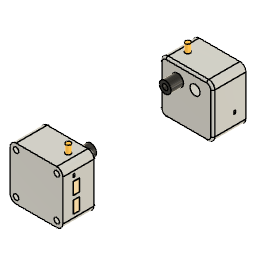
Final design 2025 project v9 (Autodesk Fusion 360 design; units mm, degrees)
Autodesk Fusion 360 part; units mm, degrees
note: some values were not read from the file. Chosen so that the rebuilt part matches the saved one: which bodies a step acts on. Set by a fixed rule: which sketch regions a step uses.
(part 1 of 2)
sketch "Sketch1" plane through (0, 0, 0) normal (0, 1, 0) x (1, 0, 0)
  line L0 (4, 0) -> (53, 0)
  line L1 (57, -4) -> (57, -53)
  line L2 (53, -57) -> (4, -57)
  line L3 (0, -53) -> (0, -4)
  circle A0 centre (18, -43.5) radius 8
  circle A1 centre (39, -43.5) radius 8
  arc A2 (0, -53) -> (4, -57) centre (4, -53) ccw
  arc A3 (53, -57) -> (57, -53) centre (53, -53) ccw
  arc A4 (57, -4) -> (53, 0) centre (53, -4) ccw
  arc A5 (4, 0) -> (0, -4) centre (4, -4) ccw
  circle A6 centre (18, -43.5) radius 2.8
  circle A7 centre (39, -43.5) radius 2.8
  circle A8 centre (4, -53) radius 1.8
  circle A9 centre (53, -53) radius 1.8
  circle A10 centre (4, -4) radius 1.8
  circle A11 centre (53, -4) radius 1.8
  line L4 (0, -8) -> (11.1, -8)
  line L5 (11.1, -8) -> (11.1, -22.6)
  line L6 (11.1, -22.6) -> (0, -22.6)
  line L7 (0, -22.6) -> (0, -8)
  line L8 (0, -27.6) -> (11.1, -27.6)
  line L9 (11.1, -27.6) -> (11.1, -42.2)
  line L10 (11.1, -42.2) -> (0, -42.2)
  line L11 (0, -42.2) -> (0, -27.6)
  line L12 (10, -57) -> (14.9, -57)
  line L13 (14.9, -57) -> (14.9, -47.5)
  line L14 (14.9, -47.5) -> (10, -47.5)
  line L15 (10, -47.5) -> (10, -57)
  line L16 (0, -49) -> (1, -49)
  line L17 (1, -49) -> (1, -47)
  line L18 (1, -47) -> (0, -47)
  line L19 (0, -47) -> (0, -49)
  arc A12 (-0.8, -53) -> (4, -57.8) centre (4, -53) ccw
  line L20 (53, -57.8) -> (4, -57.8)
  arc A13 (53, -57.8) -> (57.8, -53) centre (53, -53) ccw
  line L21 (57.8, -4) -> (57.8, -53)
  arc A14 (57.8, -4) -> (53, 0.8) centre (53, -4) ccw
  line L22 (4, 0.8) -> (53, 0.8)
  arc A15 (4, 0.8) -> (-0.8, -4) centre (4, -4) ccw
  line L23 (-0.8, -53) -> (-0.8, -4)
  arc A16 (-3.3, -53) -> (4, -60.3) centre (4, -53) ccw
  line L24 (53, -60.3) -> (4, -60.3)
  arc A17 (53, -60.3) -> (60.3, -53) centre (53, -53) ccw
  line L25 (60.3, -4) -> (60.3, -53)
  arc A18 (60.3, -4) -> (53, 3.3) centre (53, -4) ccw
  line L26 (4, 3.3) -> (53, 3.3)
  arc A19 (4, 3.3) -> (-3.3, -4) centre (4, -4) ccw
  line L27 (-3.3, -53) -> (-3.3, -4)
  arc A20 (0.6, -53) -> (4, -56.4) centre (4, -53) ccw
  line L28 (53, -56.4) -> (4, -56.4)
  arc A21 (53, -56.4) -> (56.4, -53) centre (53, -53) ccw
  line L29 (56.4, -4) -> (56.4, -53)
  arc A22 (56.4, -4) -> (53, -0.6) centre (53, -4) ccw
  line L30 (4, -0.6) -> (53, -0.6)
  arc A23 (4, -0.6) -> (0.6, -4) centre (4, -4) ccw
  line L31 (0.6, -53) -> (0.6, -4)
  arc A24 (0.8, -53) -> (4, -56.2) centre (4, -53) ccw
  line L32 (53, -56.2) -> (4, -56.2)
  arc A25 (53, -56.2) -> (56.2, -53) centre (53, -53) ccw
  line L33 (56.2, -4) -> (56.2, -53)
  arc A26 (56.2, -4) -> (53, -0.8) centre (53, -4) ccw
  line L34 (4, -0.8) -> (53, -0.8)
  arc A27 (4, -0.8) -> (0.8, -4) centre (4, -4) ccw
  line L35 (0.8, -53) -> (0.8, -4)
  line L36 (60.3, -20.1347) -> (60.3, -16.7)
  line L37 (56.2, -16.7) -> (55.2, -16.7)
  line L38 (55.2, -16.7) -> (55.2, -18.7)
  line L39 (55.2, -18.7) -> (56.2, -18.7)
  line L40 (56.2, -18.7) -> (56.2, -16.7)
  line L41 (9.43, -57) -> (13.43, -57)
  line L42 (13.43, -57) -> (13.43, -55)
  line L43 (13.43, -55) -> (9.43, -55)
  line L44 (9.43, -55) -> (9.43, -57)
  point P0 (57, 0)
  point P1 (0, -57)
  dimension "d1" = 57
  dimension "d2" = 57
  dimension "d13" = 16
  dimension "d15" = 16
  dimension "d16" = 4
  dimension "d17" = 5.6
  dimension "d18" = 5.6
  dimension "d21" = 3.6
  dimension "d22" = 3.6
  dimension "d23" = 3.6
  dimension "d24" = 3.6
  dimension "d29" = 11.1
  dimension "d30" = 11.1
  dimension "d31" = 14.6
  dimension "d34" = 4.9
  dimension "d35" = 9.5
  dimension "d37" = 1
  dimension "d38" = 2
  dimension "d40" = -0.8
  dimension "d41" = -2.5
  dimension "d58" = 0.6
  dimension "d59" = 0.8
  dimension "d61" = 1
  dimension "d62" = 2
  dimension "d65" = 4
  dimension "d66" = 2
  constraint horizontal L0
  constraint vertical L1
  constraint horizontal L2
  constraint vertical L3
  constraint coincident P1 L2
  constraint coincident P1 L3
  constraint tangent L2 A2
  constraint tangent L3 A2
  constraint tangent L1 A3
  constraint tangent L2 A3
  constraint equal A2 A3
  constraint coincident P0 L0
  constraint coincident P0 L1
  constraint tangent L0 A4
  constraint tangent L1 A4
  constraint equal A2 A4
  constraint coincident origin L0
  constraint coincident origin L3
  constraint tangent L0 A5
  constraint tangent L3 A5
  constraint equal A2 A5
  constraint concentric A0 A6
  constraint concentric A1 A7
  constraint concentric A2 A8
  constraint concentric A3 A9
  constraint concentric A5 A10
  constraint concentric A4 A11
  constraint horizontal L4
  constraint vertical L5
  constraint horizontal L6
  constraint vertical L7
  constraint horizontal L8
  constraint vertical L9
  constraint horizontal L10
  constraint vertical L11
  constraint horizontal L12
  constraint vertical L13
  constraint horizontal L14
  constraint vertical L15
  constraint coincident L2 L12.start
  constraint horizontal L16
  constraint vertical L17
  constraint horizontal L18
  constraint vertical L19
  constraint coincident L3 L16.start
  constraint vertical L36
  constraint coincident L25 L36.end
  constraint horizontal L37
  constraint vertical L38
  constraint horizontal L39
  constraint vertical L40
  constraint coincident L33 L37.start
  constraint horizontal L41
  constraint vertical L42
  constraint horizontal L43
  constraint vertical L44
  constraint coincident L2 L41.start
  measures "d1" distance of origin P0
  measures "d2" distance of origin P1
  measures "d13" diameter of A0
  measures "d15" diameter of A1
  measures "d16" radius of A2
  measures "d17" diameter of A6
  measures "d18" diameter of A7
  measures "d21" diameter of A8
  measures "d22" diameter of A9
  measures "d23" diameter of A10
  measures "d24" diameter of A11
  measures "d29" distance of L4.start L4.end
  measures "d30" distance of L8.start L8.end
  measures "d31" distance of L8.start L10.end
  measures "d34" distance of L12.start L12.end
  measures "d35" distance of L12.start L14.end
  measures "d37" distance of L16.start L16.end
  measures "d38" distance of L16.start L18.end
  measures "d61" distance of L37.start L37.end
  measures "d62" distance of L37.start L39.end
  measures "d65" distance of L41.start L41.end
  measures "d66" distance of L41.start L43.end
extrude "Extrude7" add sketch "Sketch1" along normal blind 1 contours L0 L1 L2 L3 A3 A4 A5 L4 L13 L28 A21 L29 A22 L30 A23 L31 | L3 L6 L8 L31 | L4 L13 L28 A21 L29 A22 L30 A23 L31 L32 A25 L33 A26 L34 A27 L35 L40 | L4 L6 L31 L35 | L6 L8 L31 L35 | A0 L4 L5 L6 L8 L9 L13 L32 A25 L33 A26 L34 A27 L35 L37 L38 L39 | L4 L5 L6 L35 | L2 L12 L13 L28 L42 | L3 L10 L18 L31 | L8 L10 L31 L35 | L13 L28 L32 L42 | L10 L18 L31 L35 | A0 L8 L9 L10 L35 | L15 L28 L32 L42 | A0 L13 L14 L15 L32 L42 L43 | L2 L3 A2 L16 A20 L28 L31 L44 | A0 L10 L14 L15 L16 L17 L18 A24 L32 L35 L43 L44 | L15 L28 L32 L44 | L15 L32 L42 L43 | L16 A20 L28 L31 A24 L32 L35 L44 | L16 L17 L18 L35 | L15 L32 L43 L44 makes body 1
extrude "Extrude8" cut 1 faces at (56.2, 0.3333, 17.3667) along direction (1, 0, 0) blind 10 on bodies 1 bodies 1
extrude "Extrude9" add sketch "Sketch1" along normal blind 15 separate body contours A16 L24 A17 L25 A18 L26 A19 L27 L36 makes body 2
extrude "Extrude10" add sketch "Sketch1" against normal blind 25 separate body contours A16 L24 A17 L25 A18 L26 A19 L27 L36 makes body 3
sketch "Sketch4" plane through (0, -25, 0) normal (0, -1, 0) x (1, 0, 0)
  arc A0 (57.8, 53) -> (53, 57.8) centre (53, 53) ccw
  line L0 (57.8, 53) -> (57.8, 4)
  arc A1 (53, -0.8) -> (57.8, 4) centre (53, 4) ccw
  line L1 (53, -0.8) -> (4, -0.8)
  arc A2 (-0.8, 4) -> (4, -0.8) centre (4, 4) ccw
  line L2 (-0.8, 4) -> (-0.8, 53)
  arc A3 (4, 57.8) -> (-0.8, 53) centre (4, 53) ccw
  line L3 (4, 57.8) -> (53, 57.8)
  arc A4 (60.3, 53) -> (53, 60.3) centre (53, 53) ccw
  line L4 (53, 60.3) -> (4, 60.3)
  arc A5 (4, 60.3) -> (-3.3, 53) centre (4, 53) ccw
  line L5 (-3.3, 53) -> (-3.3, 4)
  arc A6 (-3.3, 4) -> (4, -3.3) centre (4, 4) ccw
  line L6 (4, -3.3) -> (53, -3.3)
  arc A7 (53, -3.3) -> (60.3, 4) centre (53, 4) ccw
  line L7 (60.3, 4) -> (60.3, 53)
extrude "Extrude11" add sketch "Sketch4" along normal blind 2.5 bodies 3
sketch "Sketch5" plane through (0, -27.5, 0) normal (0, -1, 0) x (1, 0, 0)
  arc A0 (-0.8, 4) -> (4, -0.8) centre (4, 4) ccw
  line L0 (-0.8, 4) -> (-0.8, 53)
  arc A1 (4, 57.8) -> (-0.8, 53) centre (4, 53) ccw
  line L1 (4, 57.8) -> (53, 57.8)
  arc A2 (57.8, 53) -> (53, 57.8) centre (53, 53) ccw
  line L2 (57.8, 53) -> (57.8, 4)
  arc A3 (53, -0.8) -> (57.8, 4) centre (53, 4) ccw
  line L3 (53, -0.8) -> (4, -0.8)
  line L4 (60.3, 4) -> (60.3, 53)
  arc A4 (60.3, 53) -> (53, 60.3) centre (53, 53) ccw
  line L5 (53, 60.3) -> (4, 60.3)
  arc A5 (4, 60.3) -> (-3.3, 53) centre (4, 53) ccw
  line L6 (-3.3, 53) -> (-3.3, 4)
  arc A6 (-3.3, 4) -> (4, -3.3) centre (4, 4) ccw
  line L7 (4, -3.3) -> (53, -3.3)
  arc A7 (53, -3.3) -> (60.3, 4) centre (53, 4) ccw
extrude "Extrude12" add sketch "Sketch5" against normal blind 2.5 contours A0 L0 A1 L1 A2 L2 A3 L3 bodies 3
extrude "Extrude13" cut sketch "Sketch1" against normal blind 41 contours A0 L9 L10 L13 L14 | A0 L13 L14 | A0 L9 L10 | A1 bodies 3 makes body 4 at (41.7861, -25.8333, 43.7788) makes body 5 at (31.0258, -27.5, 9.8177)
extrude "Extrude14" cut 1 faces at (17.5333, -27.5, 44.3083) along direction (0, 1, 0) blind 6 on bodies 3 bodies 3
extrude "Extrude15" cut 1 faces at (58.6333, 15, 24.5667) along direction (0, -1, 0) blind 5 on bodies 2 bodies 2
sketch "Sketch6" plane through (0, -27.5, 0) normal (0, -1, 0) x (1, 0, 0)
  circle A0 centre (18, 43.5) radius 8
  circle A1 centre (39, 43.5) radius 8
  line L0 (60.3, 4) -> (60.3, 53)
  arc A2 (60.3, 53) -> (53, 60.3) centre (53, 53) ccw
  line L1 (53, 60.3) -> (4, 60.3)
  arc A3 (4, 60.3) -> (-3.3, 53) centre (4, 53) ccw
  line L2 (-3.3, 53) -> (-3.3, 4)
  arc A4 (-3.3, 4) -> (4, -3.3) centre (4, 4) ccw
  line L3 (4, -3.3) -> (53, -3.3)
  arc A5 (53, -3.3) -> (60.3, 4) centre (53, 4) ccw
  circle A6 centre (18, 43.5) radius 7
  dimension "d85" = 14
  constraint concentric A0 A6
  measures "d85" diameter of A6
extrude "Extrude16" add sketch "Sketch6" against normal blind 2.5 contours A0 bodies 3 5
fillet "Fillet3" radius 2.5 8 edges at (-1.1619, -27.5, -1.1619) (28.5, -27.5, -3.3) (58.1619, -27.5, -1.1619) (60.3, -27.5, 28.5) (58.1619, -27.5, 58.1619) (28.5, -27.5, 60.3) (-1.1619, -27.5, 58.1619) (-3.3, -27.5, 28.5) on bodies 3
sketch "Sketch7" plane through (0, -27.5, 0) normal (0, -1, 0) x (1, 0, 0)
  circle A0 centre (39, 43.5) radius 8
  circle A1 centre (18, 43.5) radius 7
  arc A2 (-0.8, 4) -> (4, -0.8) centre (4, 4) ccw
  line L0 (4, -0.8) -> (53, -0.8)
  arc A3 (53, -0.8) -> (57.8, 4) centre (53, 4) ccw
  line L1 (57.8, 4) -> (57.8, 53)
  arc A4 (57.8, 53) -> (53, 57.8) centre (53, 53) ccw
  line L2 (53, 57.8) -> (4, 57.8)
  arc A5 (4, 57.8) -> (-0.8, 53) centre (4, 53) ccw
  line L3 (-0.8, 53) -> (-0.8, 4)
extrude "Extrude17" add sketch "Sketch7" along normal blind 2 contours A0 bodies 3 4
extrude "Extrude18" cut 1 faces at (38.9303, -25, 44.3069) along direction (0, -1, 0) blind 14 on bodies 3 bodies 3
extrude "Extrude19" add 1 faces at (45.2265, -27.5, 44.0366) along direction (0, 1, 0) blind 2.5 on bodies 3 bodies 3
extrude "Extrude20" cut 1 faces at (45.2369, -29.5, 43.1026) along direction (0, 1, 0) blind 2 on bodies 3 bodies 3
fillet "Fillet4" radius 2.5 8 edges at (28.5, -25, 57.8) (0.6059, -25, 56.3941) (-0.8, -25, 28.5) (0.6059, -25, 0.6059) (28.5, -25, -0.8) (56.3941, -25, 0.6059) (57.8, -25, 28.5) (56.3941, -25, 56.3941) on bodies 3
sketch "Sketch8" plane through (0, -25, 0) normal (0, 1, 0) x (-1, 0, 0)
  circle A0 centre (-18, 43.5) radius 7
  circle A1 centre (-39, 43.5) radius 2.8
  line L0 (-4, 55.3) -> (-53, 55.3)
  arc A2 (-53, 55.3) -> (-55.3, 53) centre (-53, 53) ccw
  line L1 (-55.3, 53) -> (-55.3, 4)
  arc A3 (-55.3, 4) -> (-53, 1.7) centre (-53, 4) ccw
  line L2 (-53, 1.7) -> (-4, 1.7)
  arc A4 (-4, 1.7) -> (-1.7, 4) centre (-4, 4) ccw
  line L3 (-1.7, 4) -> (-1.7, 53)
  arc A5 (-1.7, 53) -> (-4, 55.3) centre (-4, 53) ccw
  circle A6 centre (-18, 43.5) radius 10
  dimension "d100" = 20
  constraint concentric A0 A6
  measures "d100" diameter of A6
extrude "Extrude21" cut sketch "Sketch8" against normal blind 0.5 contours A6 bodies 3
sketch "Sketch9" plane through (0, -25, 0) normal (0, 1, 0) x (-1, 0, 0)
  circle A0 centre (-18, 43.5) radius 10
  circle A1 centre (-39, 43.5) radius 2.8
  line L0 (-4, 55.3) -> (-53, 55.3)
  arc A2 (-53, 55.3) -> (-55.3, 53) centre (-53, 53) ccw
  line L1 (-55.3, 53) -> (-55.3, 4)
  arc A3 (-55.3, 4) -> (-53, 1.7) centre (-53, 4) ccw
  line L2 (-53, 1.7) -> (-4, 1.7)
  arc A4 (-4, 1.7) -> (-1.7, 4) centre (-4, 4) ccw
  line L3 (-1.7, 4) -> (-1.7, 53)
  arc A5 (-1.7, 53) -> (-4, 55.3) centre (-4, 53) ccw
  circle A6 centre (-39, 43.5) radius 8
  dimension "d103" = 16
  constraint concentric A1 A6
  measures "d103" diameter of A6
extrude "Extrude22" add sketch "Sketch9" along normal blind 10 contours A6 bodies 3
sketch "Sketch10" plane through (0, -27.5, 0) normal (0, -1, 0) x (1, 0, 0)
  circle A0 centre (39, 43.5) radius 2.8
  circle A1 centre (18, 43.5) radius 7
  arc A2 (-0.8, 4) -> (4, -0.8) centre (4, 4) ccw
  line L0 (4, -0.8) -> (53, -0.8)
  arc A3 (53, -0.8) -> (57.8, 4) centre (53, 4) ccw
  line L1 (57.8, 4) -> (57.8, 53)
  arc A4 (57.8, 53) -> (53, 57.8) centre (53, 53) ccw
  line L2 (53, 57.8) -> (4, 57.8)
  arc A5 (4, 57.8) -> (-0.8, 53) centre (4, 53) ccw
  line L3 (-0.8, 53) -> (-0.8, 4)
  circle A6 centre (39, 43.5) radius 6
  dimension "d106" = 12
  constraint concentric A0 A6
  measures "d106" diameter of A6
extrude "Extrude23" cut sketch "Sketch10" against normal blind 18 contours A6 bodies 3
sketch "Sketch11" plane through (0, -15, 0) normal (0, 1, 0) x (-1, 0, 0)
  circle A0 centre (-39, 43.5) radius 6
  circle A1 centre (-39, 43.5) radius 8
extrude "Extrude24" add sketch "Sketch11" against normal blind 2.5 contours A0 bodies 3
sketch "Sketch12" plane through (0, -17.5, 0) normal (0, -1, 0) x (1, 0, 0)
  circle A0 centre (39, 43.5) radius 6
  circle A1 centre (39, 43.5) radius 3.75
  dimension "d111" = 7.5
  constraint concentric A0 A1
  measures "d111" diameter of A1
extrude "Extrude25" cut sketch "Sketch12" against normal blind 11 contours A1 bodies 3
fillet "Fillet5" radius 5.5 1 edges at (33.406, -17.5, 45.6697) on bodies 3
extrude "Extrude26" cut 1 faces at (0.8, 0.3333, 48.3333) along direction (-1, 0, 0) blind 8 on bodies 1 bodies 2
extrude "Extrude27" cut 1 faces at (55.2, 0.3333, 17.3667) along direction (1, 0, 0) blind 8.5 on bodies 1 bodies 2
extrude "Extrude28" cut 1 faces at (12.0967, 0.3333, 56.4) along direction (0, 0, 1) blind 8.5 on bodies 1 bodies 2
extrude "Extrude29" cut 2 faces at (0.6, 0.6667, 37.3333) (0.6, 0.3333, 17.7333) along direction (-1, 0, 0) blind 15 on bodies 1 bodies 2
sketch "Sketch13" plane through (60.3, 0, 0) normal (1, 0, 0) x (0, 1, 0)
  line L0 (1, 16.7) -> (0, 16.7)
  line L1 (0, 16.7) -> (0, 4)
  line L2 (0, 4) -> (10, 4)
  line L3 (10, 4) -> (10, 53)
  line L4 (10, 53) -> (0, 53)
  line L5 (0, 53) -> (0, 18.7)
  line L6 (0, 18.7) -> (1, 18.7)
  line L7 (1, 18.7) -> (1, 16.7)
  line L8 (0, 18.7) -> (-1.5, 18.7)
  line L9 (-1.5, 18.7) -> (-1.5, 16.7)
  line L10 (-1.5, 16.7) -> (0, 16.7)
  line L11 (0, 16.7) -> (0, 18.7)
  circle A0 centre (0, 16.7) radius 0.75
  line L12 (0, 16.7) -> (0, 15)
  line L13 (0, 15.95) -> (-2, 15.95)
  line L14 (-2, 15.95) -> (-2, 19.45)
  line L15 (-2, 19.45) -> (0, 19.45)
  line L16 (0, 19.45) -> (0, 15.95)
  dimension "d124" = 1.5
  dimension "d125" = 1.5
  dimension "d126" = 2
  dimension "d127" = 3.5
  constraint horizontal L8
  constraint vertical L9
  constraint horizontal L10
  constraint vertical L11
  constraint coincident L5.end L6.start
  constraint coincident L0.end L1.start
  constraint coincident L1 L12.end
  constraint horizontal L13
  constraint vertical L14
  constraint horizontal L15
  constraint vertical L16
  constraint coincident L12 L13.start
  constraint coincident A0 L13.start
  measures "d124" distance of L5.end L8.end
  measures "d125" diameter of A0
  measures "d126" distance of L13.start L13.end
  measures "d127" distance of L13.start L15.end
extrude "Extrude30" cut sketch "Sketch13" against normal blind 5 contours L1 L10 A0 L12 L16 | L10 L11 A0 L16 | L5 L8 L9 L10 A0 L13 L14 L15 L16 | L8 L9 L10 L11 A0 L16 bodies 3
extrude "Extrude31" add 1 faces at (59.4667, 1, 17.3667) along direction (0, -1, 0) blind 1 on bodies 2 bodies 2
sketch "Sketch14" plane through (-3.3, 0, 0) normal (-1, 0, 0) x (0, -1, 0)
  line L0 (0, 27.6) -> (-1, 27.6)
  line L1 (-1, 27.6) -> (-1, 42.2)
  line L2 (-1, 42.2) -> (0, 42.2)
  line L3 (0, 42.2) -> (0, 47)
  line L4 (0, 47) -> (-1, 47)
  line L5 (-1, 47) -> (-1, 49)
  line L6 (-1, 49) -> (0, 49)
  line L7 (0, 49) -> (0, 53)
  line L8 (0, 53) -> (-10, 53)
  line L9 (-10, 53) -> (-10, 4)
  line L10 (-10, 4) -> (0, 4)
  line L11 (0, 4) -> (0, 8)
  line L12 (0, 8) -> (-1, 8)
  line L13 (-1, 8) -> (-1, 22.6)
  line L14 (-1, 22.6) -> (0, 22.6)
  line L15 (0, 22.6) -> (0, 27.6)
  circle A0 centre (0, 48) radius 1.75
  line L16 (0, 46.25) -> (2, 46.25)
  line L17 (2, 46.25) -> (2, 49.75)
  line L18 (2, 49.75) -> (0, 49.75)
  line L19 (0, 49.75) -> (0, 46.25)
  dimension "d132" = 3.5
  dimension "d133" = 2
  dimension "d134" = 3.5
  constraint horizontal L16
  constraint vertical L17
  constraint horizontal L18
  constraint vertical L19
  constraint coincident A0 L16.start
  constraint coincident L3 L16.start
  measures "d132" diameter of A0
  measures "d133" distance of L16.start L16.end
  measures "d134" distance of L16.start L18.end
extrude "Extrude32" cut sketch "Sketch14" against normal blind 9.5 contours L3 L7 A0 L19 | A0 L16 L17 L18 bodies 3
extrude "Extrude33" add 1 faces at (-1.6333, 1, 48.3333) along direction (0, -1, 0) blind 1 on bodies 2 bodies 2
sketch "Sketch15" plane through (-3.3, 0, 0) normal (-1, 0, 0) x (0, -1, 0)
  line L0 (0, 27.6) -> (-1, 27.6)
  line L1 (-1, 27.6) -> (-1, 42.2)
  line L2 (-1, 42.2) -> (0, 42.2)
  line L3 (0, 42.2) -> (0, 53)
  line L4 (0, 53) -> (-10, 53)
  line L5 (-10, 53) -> (-10, 4)
  line L6 (-10, 4) -> (0, 4)
  line L7 (0, 4) -> (0, 8)
  line L8 (0, 8) -> (-1, 8)
  line L9 (-1, 8) -> (-1, 22.6)
  line L10 (-1, 22.6) -> (0, 22.6)
  line L11 (0, 22.6) -> (0, 27.6)
  line L12 (0, 27.6) -> (7.6, 27.6)
  line L13 (7.6, 27.6) -> (7.6, 42.2)
  line L14 (7.6, 42.2) -> (0, 42.2)
  line L15 (0, 42.2) -> (0, 27.6)
  line L16 (0, 8) -> (7.5, 8)
  line L17 (7.5, 8) -> (7.5, 22.6)
  line L18 (7.5, 22.6) -> (0, 22.6)
  line L19 (0, 22.6) -> (0, 8)
  dimension "d139" = 7.6
  dimension "d140" = 14.6
  dimension "d141" = 7.5
  constraint horizontal L12
  constraint vertical L13
  constraint horizontal L14
  constraint vertical L15
  constraint coincident L0.start L11.end
  constraint horizontal L16
  constraint vertical L17
  constraint horizontal L18
  constraint vertical L19
  constraint coincident L7.end L8.start
  measures "d139" distance of L0.start L12.end
  measures "d140" distance of L0.start L2.end
  measures "d141" distance of L7.end L16.end
extrude "Extrude34" cut sketch "Sketch15" against normal blind 8 contours L12 L13 L14 L15 | L16 L17 L18 L19 bodies 3
sketch "Sketch16" plane through (0, 0, 60.3) normal (0, 0, 1) x (-1, 0, 0)
  line L0 (-53, 0) -> (-4, 0)
sketch "Sketch17" plane through (0, 0, 60.3) normal (0, 0, 1) x (-1, 0, 0)
  line L0 (-9.43, 0) -> (-9.43, -1)
  line L1 (-9.43, -1) -> (-13.43, -1)
  line L2 (-13.43, -1) -> (-13.43, 0)
  line L3 (-13.43, 0) -> (-53, 0)
  line L4 (-53, 0) -> (-53, -10)
  line L5 (-53, -10) -> (-4, -10)
  line L6 (-4, -10) -> (-4, 0)
  line L7 (-4, 0) -> (-9.43, 0)
  line L8 (-9.43, 0) -> (-13.43, 0)
  line L9 (-13.43, 8.81) -> (-9.43, 8.81)
  line L10 (-9.43, 8.81) -> (-9.43, 0)
  circle A0 centre (-11.43, 8.81) radius 3
  dimension "d144" = 4
  dimension "d145" = 8.81
  dimension "d146" = 6
  constraint horizontal L8
  constraint horizontal L9
  constraint vertical L10
  constraint coincident L0.start L7.end
  constraint midpoint L9 A0.centre
  measures "d144" distance of L0.start L2.end
  measures "d145" distance of L0.start L9.end
  measures "d146" diameter of A0
extrude "Extrude35" cut sketch "Sketch17" against normal blind 4 contours A0 bodies 3
move_body "Move1" bodies 3 to x (1, 0, 0) y (0, 1, 0) z (0, 0, 1) at (0, -50, 0)
extrude "Extrude36" add 1 faces at (-2.4667, 1, 37.3333) along direction (0, -1, 0) blind 1 on bodies 2 bodies 2
extrude "Extrude37" add 1 faces at (-2.4667, 1, 17.7333) along direction (0, -1, 0) blind 1 on bodies 2 bodies 2
extrude "Extrude38" add 1 faces at (10.7633, 1, 58.6333) along direction (0, -1, 0) blind 1 on bodies 2 bodies 2
sketch "Sketch18" plane through (0, 10, 0) normal (0, 1, 0) x (-1, 0, 0)
  arc A0 (-53, 57.8) -> (-57.8, 53) centre (-53, 53) ccw
  line L0 (-53, 57.8) -> (-4, 57.8)
  arc A1 (0.8, 53) -> (-4, 57.8) centre (-4, 53) ccw
  line L1 (0.8, 53) -> (0.8, 4)
  arc A2 (-4, -0.8) -> (0.8, 4) centre (-4, 4) ccw
  line L2 (-4, -0.8) -> (-53, -0.8)
  arc A3 (-57.8, 4) -> (-53, -0.8) centre (-53, 4) ccw
  line L3 (-57.8, 4) -> (-57.8, 53)
  arc A4 (-53, 60.3) -> (-60.3, 53) centre (-53, 53) ccw
  line L4 (-60.3, 53) -> (-60.3, 4)
  arc A5 (-60.3, 4) -> (-53, -3.3) centre (-53, 4) ccw
  line L5 (-53, -3.3) -> (-4, -3.3)
  arc A6 (-4, -3.3) -> (3.3, 4) centre (-4, 4) ccw
  line L6 (3.3, 4) -> (3.3, 53)
  arc A7 (3.3, 53) -> (-4, 60.3) centre (-4, 53) ccw
  line L7 (-4, 60.3) -> (-53, 60.3)
extrude "Extrude39" add sketch "Sketch18" along normal blind 2.5 contours A0 L0 A1 L1 A2 L2 A3 L3 | A4 L4 A5 L5 A6 L6 A7 L7 bodies 2
sketch "Sketch19" plane through (0, 10, 0) normal (0, -1, 0) x (1, 0, 0)
  line L0 (-0.8, 53) -> (-0.8, 4)
  arc A0 (-0.8, 4) -> (4, -0.8) centre (4, 4) ccw
  line L1 (4, -0.8) -> (53, -0.8)
  arc A1 (53, -0.8) -> (57.8, 4) centre (53, 4) ccw
  line L2 (57.8, 4) -> (57.8, 53)
  arc A2 (57.8, 53) -> (53, 57.8) centre (53, 53) ccw
  line L3 (53, 57.8) -> (4, 57.8)
  arc A3 (4, 57.8) -> (-0.8, 53) centre (4, 53) ccw
  line L4 (57.8, 53) -> (53, 53)
  line L5 (53, 53) -> (53, 57.8)
  line L6 (53, 57.8) -> (57.8, 57.8)
  line L7 (57.8, 57.8) -> (57.8, 53)
  line L8 (57.8, 57.8) -> (49.8, 57.8)
  line L9 (49.8, 57.8) -> (49.8, 49.8)
  line L10 (49.8, 49.8) -> (57.8, 49.8)
  line L11 (57.8, 49.8) -> (57.8, 57.8)
  line L12 (-0.8, 53) -> (4, 53)
  line L13 (4, 53) -> (4, 57.8)
  line L14 (4, 57.8) -> (-0.8, 57.8)
  line L15 (-0.8, 57.8) -> (-0.8, 53)
  line L16 (-0.8, 57.8) -> (7.2, 57.8)
  line L17 (7.2, 57.8) -> (7.2, 49.8)
  line L18 (7.2, 49.8) -> (-0.8, 49.8)
  line L19 (-0.8, 49.8) -> (-0.8, 57.8)
  line L20 (4, -0.8) -> (-0.8, -0.8)
  line L21 (-0.8, -0.8) -> (-0.8, 4)
  line L22 (-0.8, 4) -> (4, 4)
  line L23 (4, 4) -> (4, -0.8)
  line L24 (-0.8, -0.8) -> (7.2, -0.8)
  line L25 (7.2, -0.8) -> (7.2, 7.2)
  line L26 (7.2, 7.2) -> (-0.8, 7.2)
  line L27 (-0.8, 7.2) -> (-0.8, -0.8)
  line L28 (53, -0.8) -> (57.8, -0.8)
  line L29 (57.8, -0.8) -> (57.8, 4)
  line L30 (57.8, 4) -> (53, 4)
  line L31 (53, 4) -> (53, -0.8)
  line L32 (57.8, -0.8) -> (49.8, -0.8)
  line L33 (49.8, -0.8) -> (49.8, 7.2)
  line L34 (49.8, 7.2) -> (57.8, 7.2)
  line L35 (57.8, 7.2) -> (57.8, -0.8)
  dimension "d157" = 8
  dimension "d158" = 8
  dimension "d159" = 8
  dimension "d160" = 8
  dimension "d161" = 8
  dimension "d162" = 8
  dimension "d163" = 8
  dimension "d164" = 8
  constraint horizontal L4
  constraint vertical L5
  constraint horizontal L6
  constraint vertical L7
  constraint coincident A2.end L3.start
  constraint coincident L2.end A2.start
  constraint horizontal L8
  constraint vertical L9
  constraint horizontal L10
  constraint vertical L11
  constraint horizontal L12
  constraint vertical L13
  constraint horizontal L14
  constraint vertical L15
  constraint coincident L3.end A3.start
  constraint coincident L0.start A3.end
  constraint horizontal L16
  constraint vertical L17
  constraint horizontal L18
  constraint vertical L19
  constraint horizontal L20
  constraint vertical L21
  constraint horizontal L22
  constraint vertical L23
  constraint coincident L0.end A0.start
  constraint coincident A0.end L1.start
  constraint horizontal L24
  constraint vertical L25
  constraint horizontal L26
  constraint vertical L27
  constraint horizontal L28
  constraint vertical L29
  constraint horizontal L30
  constraint vertical L31
  constraint coincident A1.end L2.start
  constraint coincident L1.end A1.start
  constraint horizontal L32
  constraint vertical L33
  constraint horizontal L34
  constraint vertical L35
  measures "d157" distance of L6.end L8.end
  measures "d158" distance of L6.end L10.end
  measures "d159" distance of L14.end L16.end
  measures "d160" distance of L14.end L18.end
  measures "d161" distance of L20.end L24.end
  measures "d162" distance of L20.end L26.end
  measures "d163" distance of L28.end L32.end
  measures "d164" distance of L28.end L34.end
extrude "Extrude40" add sketch "Sketch19" along normal blind 8.75 contours L0 L3 L12 L13 L16 L17 L18 L19 | A3 L12 L13 | L0 L1 L22 L23 L24 L25 L26 L27 | A0 L22 L23 | L2 L3 L4 L5 L8 L9 L10 L11 | A2 L4 L5 | L1 L2 L30 L31 L32 L33 L34 L35 | A1 L30 L31 bodies 2
sketch "Sketch20" plane through (0, -50, 0) normal (0, 1, 0) x (-1, 0, 0)
  line L0 (0.8, 49.75) -> (3.3, 49.75)
  line L1 (3.3, 49.75) -> (3.3, 53)
  arc A0 (3.3, 53) -> (-4, 60.3) centre (-4, 53) ccw
  line L2 (-4, 60.3) -> (-53, 60.3)
  arc A1 (-53, 60.3) -> (-60.3, 53) centre (-53, 53) ccw
  line L3 (-60.3, 53) -> (-60.3, 19.45)
  line L4 (-60.3, 19.45) -> (-57.8, 19.45)
  line L5 (-57.8, 19.45) -> (-57.8, 53)
  arc A2 (-53, 57.8) -> (-57.8, 53) centre (-53, 53) ccw
  line L6 (-53, 57.8) -> (-4, 57.8)
  arc A3 (0.8, 53) -> (-4, 57.8) centre (-4, 53) ccw
  line L7 (0.8, 53) -> (0.8, 49.75)
  line L8 (-4, 57.8) -> (0.8, 57.8)
  line L9 (0.8, 57.8) -> (0.8, 53)
  line L10 (0.8, 53) -> (-4, 53)
  line L11 (-4, 53) -> (-4, 57.8)
  line L12 (0.8, 57.8) -> (-7.2, 57.8)
  line L13 (-7.2, 57.8) -> (-7.2, 49.8)
  line L14 (-7.2, 49.8) -> (0.8, 49.8)
  line L15 (0.8, 49.8) -> (0.8, 57.8)
  line L16 (-57.8, 53) -> (-53, 53)
  line L17 (-53, 53) -> (-53, 57.8)
  line L18 (-53, 57.8) -> (-57.8, 57.8)
  line L19 (-57.8, 57.8) -> (-57.8, 53)
  line L20 (-57.8, 57.8) -> (-49.8, 57.8)
  line L21 (-49.8, 57.8) -> (-49.8, 49.8)
  line L22 (-49.8, 49.8) -> (-57.8, 49.8)
  line L23 (-57.8, 49.8) -> (-57.8, 57.8)
  dimension "d167" = 8
  dimension "d168" = 8
  dimension "d169" = 8
  dimension "d170" = 8
  constraint horizontal L8
  constraint vertical L9
  constraint horizontal L10
  constraint vertical L11
  constraint coincident A3.start L7.start
  constraint coincident L6.end A3.end
  constraint horizontal L12
  constraint vertical L13
  constraint horizontal L14
  constraint vertical L15
  constraint horizontal L16
  constraint vertical L17
  constraint horizontal L18
  constraint vertical L19
  constraint coincident A2.start L6.start
  constraint coincident L5.end A2.end
  constraint horizontal L20
  constraint vertical L21
  constraint horizontal L22
  constraint vertical L23
  measures "d167" distance of L8.end L12.end
  measures "d168" distance of L8.end L14.end
  measures "d169" distance of L18.end L20.end
  measures "d170" distance of L18.end L22.end
extrude "Extrude41" add sketch "Sketch20" against normal blind 26 contours L6 L7 L10 L11 L12 L13 L14 L15 | A3 L10 L11 | L5 L6 L16 L17 L20 L21 L22 L23 | A2 L16 L17 bodies 3
sketch "Sketch21" plane through (0, -50, 0) normal (0, 1, 0) x (-1, 0, 0)
  line L0 (3.3, 8) -> (0.8, 8)
  line L1 (0.8, 8) -> (0.8, 4)
  arc A0 (-4, -0.8) -> (0.8, 4) centre (-4, 4) ccw
  line L2 (-4, -0.8) -> (-53, -0.8)
  arc A1 (-57.8, 4) -> (-53, -0.8) centre (-53, 4) ccw
  line L3 (-57.8, 4) -> (-57.8, 15.95)
  line L4 (-57.8, 15.95) -> (-60.3, 15.95)
  line L5 (-60.3, 15.95) -> (-60.3, 4)
  arc A2 (-60.3, 4) -> (-53, -3.3) centre (-53, 4) ccw
  line L6 (-53, -3.3) -> (-4, -3.3)
  arc A3 (-4, -3.3) -> (3.3, 4) centre (-4, 4) ccw
  line L7 (3.3, 4) -> (3.3, 8)
  line L8 (-53, -0.8) -> (-57.8, -0.8)
  line L9 (-57.8, -0.8) -> (-57.8, 4)
  line L10 (-57.8, 4) -> (-53, 4)
  line L11 (-53, 4) -> (-53, -0.8)
  line L12 (-57.8, -0.8) -> (-49.8, -0.8)
  line L13 (-49.8, -0.8) -> (-49.8, 7.2)
  line L14 (-49.8, 7.2) -> (-57.8, 7.2)
  line L15 (-57.8, 7.2) -> (-57.8, -0.8)
  line L16 (-3.7758, -0.8) -> (0.8, -0.8)
  line L17 (0.8, -0.8) -> (0.8, 4)
  line L18 (0.8, 4) -> (-3.7758, 4)
  line L19 (-3.7758, 4) -> (-3.7758, -0.8)
  line L20 (0.8, -0.8) -> (-7.2, -0.8)
  line L21 (-7.2, -0.8) -> (-7.2, 7.2)
  line L22 (-7.2, 7.2) -> (0.8, 7.2)
  line L23 (0.8, 7.2) -> (0.8, -0.8)
  dimension "d173" = 8
  dimension "d174" = 8
  dimension "d175" = 8
  dimension "d176" = 8
  constraint horizontal L8
  constraint vertical L9
  constraint horizontal L10
  constraint vertical L11
  constraint coincident A1.start L3.start
  constraint coincident L2.end A1.end
  constraint horizontal L12
  constraint vertical L13
  constraint horizontal L14
  constraint vertical L15
  constraint horizontal L16
  constraint vertical L17
  constraint horizontal L18
  constraint vertical L19
  constraint coincident L1.end A0.end
  constraint horizontal L20
  constraint vertical L21
  constraint horizontal L22
  constraint vertical L23
  measures "d173" distance of L8.end L12.end
  measures "d174" distance of L8.end L14.end
  measures "d175" distance of L16.end L20.end
  measures "d176" distance of L16.end L22.end
extrude "Extrude42" add sketch "Sketch21" against normal blind 26 contours L1 A0 L2 L18 L19 L20 L21 L22 L23 | A0 L18 L19 | L2 L3 L10 L11 L12 L13 L14 L15 | A1 L10 L11 bodies 3
sketch "Sketch22" plane through (0, 10, 0) normal (0, -1, 0) x (1, 0, 0)
  line L0 (49.8, 7.2) -> (57.8, 7.2)
  line L1 (57.8, 7.2) -> (57.8, 49.8)
  line L2 (57.8, 49.8) -> (49.8, 49.8)
  line L3 (49.8, 49.8) -> (49.8, 57.8)
  line L4 (49.8, 57.8) -> (7.2, 57.8)
  line L5 (7.2, 57.8) -> (7.2, 49.8)
  line L6 (7.2, 49.8) -> (-0.8, 49.8)
  line L7 (-0.8, 49.8) -> (-0.8, 7.2)
  line L8 (-0.8, 7.2) -> (7.2, 7.2)
  line L9 (7.2, 7.2) -> (7.2, -0.8)
  line L10 (7.2, -0.8) -> (49.8, -0.8)
  line L11 (49.8, -0.8) -> (49.8, 7.2)
  line L12 (-0.8, 49.8) -> (1.2, 49.8)
  line L13 (1.2, 49.8) -> (1.2, 7.2302)
  line L14 (1.2, 7.2302) -> (-0.8, 7.2302)
  line L15 (-0.8, 7.2302) -> (-0.8, 49.8)
  line L16 (49.8, -0.8) -> (7.2, -0.8)
  line L17 (7.2, -0.8) -> (7.2, 1.2)
  line L18 (7.2, 1.2) -> (49.8, 1.2)
  line L19 (49.8, 1.2) -> (49.8, -0.8)
  line L20 (57.8, 7.2) -> (55.8, 7.2)
  line L21 (55.8, 7.2) -> (55.8, 49.8)
  line L22 (55.8, 49.8) -> (57.8, 49.8)
  line L23 (57.8, 49.8) -> (57.8, 7.2)
  line L24 (7.2, 57.8) -> (49.8, 57.8)
  line L25 (49.8, 57.8) -> (49.8, 55.8)
  line L26 (49.8, 55.8) -> (7.2, 55.8)
  line L27 (7.2, 55.8) -> (7.2, 57.8)
  dimension "d180" = 2
  dimension "d181" = 2
  dimension "d182" = 2
  dimension "d183" = 2
  constraint horizontal L12
  constraint vertical L13
  constraint horizontal L14
  constraint vertical L15
  constraint coincident L6.end L7.start
  constraint horizontal L16
  constraint vertical L17
  constraint horizontal L18
  constraint vertical L19
  constraint coincident L10.end L11.start
  constraint horizontal L20
  constraint vertical L21
  constraint horizontal L22
  constraint vertical L23
  constraint coincident L0.end L1.start
  constraint horizontal L24
  constraint vertical L25
  constraint horizontal L26
  constraint vertical L27
  constraint coincident L3 L25.end
  constraint coincident L4.end L5.start
  measures "d180" distance of L6.end L12.end
  measures "d181" distance of L10.end L18.end
  measures "d182" distance of L0.end L20.end
  measures "d183" distance of L4.end L26.end
extrude "Extrude43" add sketch "Sketch22" along normal blind 8.75 contours L0 L1 L2 L20 L21 L22 L23 | L9 L10 L11 L16 L17 L18 L19 | L3 L4 L5 L24 L25 L26 L27 | L6 L7 L12 L13 L14 L15 bodies 2
sketch "Sketch23" plane through (0, 1.25, 0) normal (0, -1, 0) x (1, 0, 0)
  line L0 (-0.8, 7.2) -> (-0.8, 4)
  arc A0 (-0.8, 4) -> (4, -0.8) centre (4, 4) ccw
  line L1 (4, -0.8) -> (53, -0.8)
  arc A1 (53, -0.8) -> (57.8, 4) centre (53, 4) ccw
  line L2 (57.8, 4) -> (57.8, 53)
  arc A2 (57.8, 53) -> (53, 57.8) centre (53, 53) ccw
  line L3 (53, 57.8) -> (4, 57.8)
  arc A3 (4, 57.8) -> (-0.8, 53) centre (4, 53) ccw
  line L4 (-0.8, 53) -> (-0.8, 7.2302)
  line L5 (-0.8, 7.2302) -> (1.2, 7.2302)
  line L6 (1.2, 7.2302) -> (1.2, 49.8)
  line L7 (1.2, 49.8) -> (7.2, 49.8)
  line L8 (7.2, 49.8) -> (7.2, 55.8)
  line L9 (7.2, 55.8) -> (49.8, 55.8)
  line L10 (49.8, 55.8) -> (49.8, 49.8)
  line L11 (49.8, 49.8) -> (55.8, 49.8)
  line L12 (55.8, 49.8) -> (55.8, 7.2)
  line L13 (55.8, 7.2) -> (49.8, 7.2)
  line L14 (49.8, 7.2) -> (49.8, 1.2)
  line L15 (49.8, 1.2) -> (7.2, 1.2)
  line L16 (7.2, 1.2) -> (7.2, 7.2)
  line L17 (7.2, 7.2) -> (-0.8, 7.2)
  line L18 (7.2, 55.8) -> (21.9074, 55.8)
  line L19 (21.9074, 55.8) -> (21.9074, 57.8)
  line L20 (21.9074, 57.8) -> (7.2, 57.8)
  line L21 (7.2, 57.8) -> (7.2, 55.8)
  constraint horizontal L18
  constraint vertical L19
  constraint horizontal L20
  constraint vertical L21
  constraint coincident L3 L19.end
  constraint coincident L8.end L9.start
extrude "Extrude44" add 1 faces at (0.5333, 4.1667, 7.2302) along direction (0, 0, -1) blind 0.05 on bodies 2 bodies 2
extrude "Extrude45" cut sketch "Sketch23" against normal blind 6 contours L3 L9 L18 L19 L20 L21 bodies 2
sketch "Sketch24" plane through (0, 0, 0) normal (0, -1, 0) x (1, 0, 0)
  line L0 (57, 16.7) -> (55.2, 16.7)
  line L1 (55.2, 16.7) -> (55.2, 18.7)
  line L2 (55.2, 18.7) -> (57, 18.7)
  line L3 (57, 18.7) -> (57, 53)
  arc A0 (57, 53) -> (53, 57) centre (53, 53) ccw
  line L4 (53, 57) -> (13.43, 57)
  line L5 (13.43, 57) -> (13.43, 56.4)
  line L6 (13.43, 56.4) -> (9.43, 56.4)
  line L7 (9.43, 56.4) -> (9.43, 57)
  line L8 (9.43, 57) -> (4, 57)
  arc A1 (4, 57) -> (0, 53) centre (4, 53) ccw
  line L9 (0, 53) -> (0, 49)
  line L10 (0, 49) -> (0.8, 49)
  line L11 (0.8, 49) -> (0.8, 47)
  line L12 (0.8, 47) -> (0, 47)
  line L13 (0, 47) -> (0, 42.2)
  line L14 (0, 42.2) -> (0.6, 42.2)
  line L15 (0.6, 42.2) -> (0.6, 27.6)
  line L16 (0.6, 27.6) -> (0, 27.6)
  line L17 (0, 27.6) -> (0, 22.6)
  line L18 (0, 22.6) -> (0.6, 22.6)
  line L19 (0.6, 22.6) -> (0.6, 8)
  line L20 (0.6, 8) -> (0, 8)
  line L21 (0, 8) -> (0, 4)
  arc A2 (0, 4) -> (4, 0) centre (4, 4) ccw
  line L22 (4, 0) -> (53, 0)
  arc A3 (53, 0) -> (57, 4) centre (53, 4) ccw
  line L23 (57, 4) -> (57, 16.7)
  circle A4 centre (53, 4) radius 1.8
  circle A5 centre (53, 53) radius 1.8
  circle A6 centre (18, 43.5) radius 8
  circle A7 centre (4, 4) radius 1.8
  circle A8 centre (4, 53) radius 1.8
  circle A9 centre (39, 43.5) radius 8
extrude "Extrude46" cut sketch "Sketch24" along normal blind 90 and the other way blind 40 contours A4 | A5 | A7 | A8 bodies 2 3
sketch "Sketch25" plane through (0, 12.5, 0) normal (0, 1, 0) x (-1, 0, 0)
  circle A0 centre (-4, 4) radius 1.8
  circle A1 centre (-4, 53) radius 1.8
  circle A2 centre (-53, 4) radius 1.8
  circle A3 centre (-53, 53) radius 1.8
  line L0 (-4, 60.3) -> (-53, 60.3)
  arc A4 (-53, 60.3) -> (-60.3, 53) centre (-53, 53) ccw
  line L1 (-60.3, 53) -> (-60.3, 4)
  arc A5 (-60.3, 4) -> (-53, -3.3) centre (-53, 4) ccw
  line L2 (-53, -3.3) -> (-4, -3.3)
  arc A6 (-4, -3.3) -> (3.3, 4) centre (-4, 4) ccw
  line L3 (3.3, 4) -> (3.3, 53)
  arc A7 (3.3, 53) -> (-4, 60.3) centre (-4, 53) ccw
  circle A8 centre (-53, 53) radius 2.5
  dimension "d195" = 5
  constraint concentric A3 A8
  measures "d195" diameter of A8
extrude "Extrude47" cut sketch "Sketch25" against normal blind 8 contours A8 bodies 2
move_body "Move2" bodies 1 to x (1, 0, 0) y (0, 1, 0) z (0, 0, 1) at (0, -20, 0)
sketch "Sketch26" plane through (0, 12.5, 0) normal (0, 1, 0) x (-1, 0, 0)
  circle A0 centre (-4, 4) radius 1.8
  circle A1 centre (-4, 53) radius 1.8
  circle A2 centre (-53, 4) radius 1.8
  line L0 (-4, 60.3) -> (-53, 60.3)
  arc A3 (-53, 60.3) -> (-60.3, 53) centre (-53, 53) ccw
  arc A4 (-60.3, 4) -> (-53, -3.3) centre (-53, 4) ccw
  line L1 (-53, -3.3) -> (-4, -3.3)
  arc A5 (-4, -3.3) -> (3.3, 4) centre (-4, 4) ccw
  line L2 (3.3, 4) -> (3.3, 53)
  arc A6 (3.3, 53) -> (-4, 60.3) centre (-4, 53) ccw
extrude "Extrude48" add 1 faces at (50.7493, 4.5, 52.7864) along direction (0, 1, 0) blind 8 on bodies 2 bodies 2
sketch "Sketch27" plane through (0, 12.5, 0) normal (0, 1, 0) x (-1, 0, 0)
  circle A0 centre (-53, 53) radius 1.8
  circle A1 centre (-4, 4) radius 1.8
  circle A2 centre (-4, 53) radius 1.8
  circle A3 centre (-53, 4) radius 1.8
  line L0 (-4, 60.3) -> (-53, 60.3)
  arc A4 (-53, 60.3) -> (-60.3, 53) centre (-53, 53) ccw
  line L1 (-60.3, 53) -> (-60.3, 4)
  arc A5 (-60.3, 4) -> (-53, -3.3) centre (-53, 4) ccw
  line L2 (-53, -3.3) -> (-4, -3.3)
  arc A6 (-4, -3.3) -> (3.3, 4) centre (-4, 4) ccw
  line L3 (3.3, 4) -> (3.3, 53)
  arc A7 (3.3, 53) -> (-4, 60.3) centre (-4, 53) ccw
sketch "Sketch28" plane through (0, -50, 0) normal (0, 1, 0) x (-1, 0, 0)
  line L0 (3.3, 27.6) -> (0.8, 27.6)
  line L1 (0.8, 27.6) -> (0.8, 22.6)
  line L2 (0.8, 22.6) -> (3.3, 22.6)
  line L3 (3.3, 22.6) -> (3.3, 27.6)
  line L4 (0.8, 25.1) -> (-0.7, 25.1)
  line L5 (-0.7, 25.1) -> (-0.7, 23.6)
  line L6 (-0.7, 23.6) -> (0.8, 23.6)
  line L7 (0.8, 23.6) -> (0.8, 25.1)
  line L8 (0.8, 25.1) -> (-0.7, 25.1)
  line L9 (-0.7, 25.1) -> (-0.7, 26.6)
  line L10 (-0.7, 26.6) -> (0.8, 26.6)
  line L11 (0.8, 26.6) -> (0.8, 25.1)
  dimension "d202" = 1.5
  dimension "d203" = 1.5
  dimension "d204" = 1.5
  constraint horizontal L4
  constraint vertical L5
  constraint horizontal L6
  constraint vertical L7
  constraint midpoint L1 L4.start
  constraint horizontal L8
  constraint vertical L9
  constraint horizontal L10
  constraint vertical L11
  measures "d202" distance of L4.start L4.end
  measures "d203" distance of L4.start L6.end
  measures "d204" distance of L4.start L10.end
extrude "Extrude49" add sketch "Sketch28" against normal blind 26 contours L1 L4 L8 L9 L10 L11 | L1 L4 L5 L6 L7 L8 bodies 3
sketch "Sketch29" plane through (0, -77.5, 0) normal (0, -1, 0) x (1, 0, 0)
  circle A0 centre (4, 4) radius 1.8
  circle A1 centre (4, 53) radius 1.8
  circle A2 centre (53, 4) radius 1.8
  circle A3 centre (53, 53) radius 1.8
  circle A4 centre (39, 43.5) radius 6
  circle A5 centre (18, 43.5) radius 7
  arc A6 (-0.8, 4) -> (4, -0.8) centre (4, 4) ccw
  line L0 (4, -0.8) -> (53, -0.8)
  arc A7 (53, -0.8) -> (57.8, 4) centre (53, 4) ccw
  line L1 (57.8, 4) -> (57.8, 53)
  arc A8 (57.8, 53) -> (53, 57.8) centre (53, 53) ccw
  line L2 (53, 57.8) -> (4, 57.8)
  arc A9 (4, 57.8) -> (-0.8, 53) centre (4, 53) ccw
  line L3 (-0.8, 53) -> (-0.8, 4)
extrude "Extrude50" cut sketch "Sketch29" against normal blind 25 contours A4 bodies 3
sketch "Sketch30" plane through (0, -65, 0) normal (0, 1, 0) x (-1, 0, 0)
  circle A0 centre (-39, 43.5) radius 6
  circle A1 centre (-39, 43.5) radius 8
  circle A2 centre (-39, 43.5) radius 9
  dimension "d209" = 18
  constraint concentric A0 A2
  measures "d209" diameter of A2
extrude "Extrude51" add sketch "Sketch30" against normal blind 12 contours A2 bodies 3
fillet "Fillet7" radius 3 1 edges at (47.3909, -75, 46.7545) on bodies 3
sketch "Sketch31" plane through (0, 12.5, 0) normal (0, 1, 0) x (-1, 0, 0)
  circle A0 centre (-53, 53) radius 1.8
  circle A1 centre (-4, 4) radius 1.8
  circle A2 centre (-4, 53) radius 1.8
  circle A3 centre (-53, 4) radius 1.8
  line L0 (-4, 60.3) -> (-53, 60.3)
  arc A4 (-53, 60.3) -> (-60.3, 53) centre (-53, 53) ccw
  line L1 (-60.3, 53) -> (-60.3, 4)
  arc A5 (-60.3, 4) -> (-53, -3.3) centre (-53, 4) ccw
  line L2 (-53, -3.3) -> (-4, -3.3)
  arc A6 (-4, -3.3) -> (3.3, 4) centre (-4, 4) ccw
  line L3 (3.3, 4) -> (3.3, 53)
  arc A7 (3.3, 53) -> (-4, 60.3) centre (-4, 53) ccw
  circle A8 centre (-53, 53) radius 3.25
  circle A9 centre (-4, 53) radius 3.25
  circle A10 centre (-53, 4) radius 3.25
  circle A11 centre (-4, 4) radius 3.25
  dimension "d214" = 6.5
  dimension "d215" = 6.5
  dimension "d216" = 6.5
  dimension "d217" = 6.5
  constraint concentric A0 A8
  constraint concentric A2 A9
  constraint concentric A3 A10
  constraint concentric A1 A11
  measures "d214" diameter of A8
  measures "d215" diameter of A9
  measures "d216" diameter of A10
  measures "d217" diameter of A11
extrude "Extrude52" cut sketch "Sketch31" against normal blind 5 contours A8 | A9 | A10 | A11 bodies 2
extrude "Extrude53" add 1 faces at (35.6, 10, 21.4) along direction (0, -1, 0) blind 0.5 on bodies 2 bodies 2
sketch "Sketch32" plane through (0, 1.25, 0) normal (0, -1, 0) x (1, 0, 0)
  circle A0 centre (4, 4) radius 1.8
  circle A1 centre (4, 53) radius 1.8
  circle A2 centre (53, 4) radius 1.8
  circle A3 centre (53, 53) radius 1.8
  line L0 (21.9074, 57.8) -> (21.9074, 55.8)
  line L1 (21.9074, 55.8) -> (49.8, 55.8)
  line L2 (49.8, 55.8) -> (49.8, 49.8)
  line L3 (49.8, 49.8) -> (55.8, 49.8)
  line L4 (55.8, 49.8) -> (55.8, 7.2)
  line L5 (55.8, 7.2) -> (49.8, 7.2)
  line L6 (49.8, 7.2) -> (49.8, 1.2)
  line L7 (49.8, 1.2) -> (7.2, 1.2)
  line L8 (7.2, 1.2) -> (7.2, 7.2)
  line L9 (7.2, 7.2) -> (1.2, 7.2)
  line L10 (1.2, 7.2) -> (1.2, 49.8)
  line L11 (1.2, 49.8) -> (7.2, 49.8)
  line L12 (7.2, 49.8) -> (7.2, 57.8)
  line L13 (7.2, 57.8) -> (4, 57.8)
  arc A4 (4, 57.8) -> (-0.8, 53) centre (4, 53) ccw
  line L14 (-0.8, 53) -> (-0.8, 4)
  arc A5 (-0.8, 4) -> (4, -0.8) centre (4, 4) ccw
  line L15 (4, -0.8) -> (53, -0.8)
  arc A6 (53, -0.8) -> (57.8, 4) centre (53, 4) ccw
  line L16 (57.8, 4) -> (57.8, 53)
  arc A7 (57.8, 53) -> (53, 57.8) centre (53, 53) ccw
  line L17 (53, 57.8) -> (21.9074, 57.8)
  line L18 (49.8, 55.8) -> (55.8, 55.8)
  line L19 (55.8, 55.8) -> (55.8, 49.8)
  line L20 (55.8, 49.8) -> (49.8, 49.8)
  line L21 (49.8, 49.8) -> (49.8, 55.8)
  line L22 (55.8, 55.8) -> (47.3, 55.8)
  line L23 (47.3, 55.8) -> (47.3, 47.3)
  line L24 (47.3, 47.3) -> (55.8, 47.3)
  line L25 (55.8, 47.3) -> (55.8, 55.8)
  line L26 (1.2, 49.8) -> (7.2, 49.8)
  line L27 (7.2, 49.8) -> (7.2, 55.8)
  line L28 (7.2, 55.8) -> (1.2, 55.8)
  line L29 (1.2, 55.8) -> (1.2, 49.8)
  line L30 (1.2, 55.8) -> (9.7, 55.8)
  line L31 (9.7, 55.8) -> (9.7, 47.3)
  line L32 (9.7, 47.3) -> (1.2, 47.3)
  line L33 (1.2, 47.3) -> (1.2, 55.8)
  line L34 (1.2, 7.2) -> (7.2, 7.2)
  line L35 (7.2, 7.2) -> (7.2, 1.2)
  line L36 (7.2, 1.2) -> (1.2, 1.2)
  line L37 (1.2, 1.2) -> (1.2, 7.2)
  line L38 (1.2, 1.2) -> (9.7, 1.2)
  line L39 (9.7, 1.2) -> (9.7, 9.7)
  line L40 (9.7, 9.7) -> (1.2, 9.7)
  line L41 (1.2, 9.7) -> (1.2, 1.2)
  line L42 (49.8, 7.2) -> (55.8, 7.2)
  line L43 (55.8, 7.2) -> (55.8, 1.2)
  line L44 (55.8, 1.2) -> (49.8, 1.2)
  line L45 (49.8, 1.2) -> (49.8, 7.2)
  line L46 (55.8, 1.2) -> (47.3, 1.2)
  line L47 (47.3, 1.2) -> (47.3, 9.7)
  line L48 (47.3, 9.7) -> (55.8, 9.7)
  line L49 (55.8, 9.7) -> (55.8, 1.2)
  dimension "d222" = 8.5
  dimension "d223" = 8.5
  dimension "d224" = 6
  dimension "d225" = 6
  dimension "d226" = 8.5
  dimension "d227" = 8.5
  dimension "d228" = 8.5
  dimension "d229" = 8.5
  dimension "d230" = 6
  dimension "d231" = 6
  dimension "d232" = 8.5
  dimension "d233" = 8.5
  constraint horizontal L18
  constraint vertical L19
  constraint horizontal L20
  constraint vertical L21
  constraint coincident L3.end L4.start
  constraint coincident L1.end L2.start
  constraint horizontal L22
  constraint vertical L23
  constraint horizontal L24
  constraint vertical L25
  constraint horizontal L26
  constraint vertical L27
  constraint horizontal L28
  constraint vertical L29
  constraint coincident L10.end L11.start
  constraint horizontal L30
  constraint vertical L31
  constraint horizontal L32
  constraint vertical L33
  constraint horizontal L34
  constraint vertical L35
  constraint horizontal L36
  constraint vertical L37
  constraint coincident L7.end L8.start
  constraint coincident L9.end L10.start
  constraint horizontal L38
  constraint vertical L39
  constraint horizontal L40
  constraint vertical L41
  constraint horizontal L42
  constraint vertical L43
  constraint horizontal L44
  constraint vertical L45
  constraint coincident L5.end L6.start
  constraint horizontal L46
  constraint vertical L47
  constraint horizontal L48
  constraint vertical L49
  measures "d222" distance of L18.end L22.end
  measures "d223" distance of L18.end L24.end
  measures "d224" distance of L10.end L11.end
  measures "d225" distance of L10.end L28.end
  measures "d226" distance of L28.end L30.end
  measures "d227" distance of L28.end L32.end
  measures "d228" distance of L36.end L38.end
  measures "d229" distance of L36.end L40.end
  measures "d230" distance of L5.end L4.end
  measures "d231" distance of L5.end L6.end
  measures "d232" distance of L43.end L46.end
  measures "d233" distance of L43.end L48.end
extrude "Extrude54" add sketch "Sketch32" along normal blind 2 and the other way blind 9 contours L1 L2 L3 L4 L20 L21 L22 L23 L24 L25 | L4 L5 L6 L7 L42 L45 L46 L47 L48 L49 | L7 L8 L9 L10 L34 L35 L38 L39 L40 L41 | L10 L11 L12 L26 L27 L30 L31 L32 L33 bodies 2
extrude "Extrude55" cut 4 faces at (8.8667, -0.75, 6.0333) (48.1333, -0.75, 6.0333) (6.0333, -0.75, 48.1333) (50.9667, -0.75, 48.1333) along direction (0, 1, 0) blind 5 on bodies 2 bodies 2
extrude "Extrude56" add 1 faces at (12.9358, 7.25, 57.1333) along direction (0, -1, 0) blind 3 on bodies 2 bodies 2
sketch "Sketch33" plane through (0, 12.5, 0) normal (0, 1, 0) x (-1, 0, 0)
  circle A0 centre (-4, 53) radius 3.25
  circle A1 centre (-4, 4) radius 3.25
  circle A2 centre (-53, 53) radius 3.25
  circle A3 centre (-53, 4) radius 3.25
  line L0 (-4, 60.3) -> (-53, 60.3)
  arc A4 (-53, 60.3) -> (-60.3, 53) centre (-53, 53) ccw
  line L1 (-60.3, 53) -> (-60.3, 4)
  arc A5 (-60.3, 4) -> (-53, -3.3) centre (-53, 4) ccw
  line L2 (-53, -3.3) -> (-4, -3.3)
  arc A6 (-4, -3.3) -> (3.3, 4) centre (-4, 4) ccw
  line L3 (3.3, 4) -> (3.3, 53)
  arc A7 (3.3, 53) -> (-4, 60.3) centre (-4, 53) ccw
extrude "Extrude57" cut sketch "Sketch33" against normal blind 5 contours A0 | A1 | A2 | A3 bodies 2
sketch "Sketch34" plane through (0, -50, 0) normal (0, 1, 0) x (-1, 0, 0)
  circle A0 centre (-4, 53) radius 1.8
  circle A1 centre (-53, 53) radius 1.8
  line L0 (0.8, 49.75) -> (3.3, 49.75)
  line L1 (3.3, 49.75) -> (3.3, 53)
  arc A2 (3.3, 53) -> (-4, 60.3) centre (-4, 53) ccw
  line L2 (-4, 60.3) -> (-53, 60.3)
  arc A3 (-53, 60.3) -> (-60.3, 53) centre (-53, 53) ccw
  line L3 (-60.3, 53) -> (-60.3, 19.45)
  line L4 (-60.3, 19.45) -> (-57.8, 19.45)
  line L5 (-57.8, 19.45) -> (-57.8, 49.8)
  line L6 (-57.8, 49.8) -> (-49.8, 49.8)
  line L7 (-49.8, 49.8) -> (-49.8, 57.8)
  line L8 (-49.8, 57.8) -> (-7.2, 57.8)
  line L9 (-7.2, 57.8) -> (-7.2, 49.8)
  line L10 (-7.2, 49.8) -> (0.8, 49.8)
  line L11 (0.8, 49.8) -> (0.8, 49.75)
  circle A4 centre (-4, 53) radius 3.1
  line L12 (-4, 53) -> (-0.9, 53)
  line L13 (-0.9, 53) -> (-0.9, 56.1)
  line L14 (-0.9, 56.1) -> (-4, 56.1)
  line L15 (-4, 56.1) -> (-4, 53)
  line L16 (-0.9, 56.1) -> (-7.1, 56.1)
  line L17 (-7.1, 56.1) -> (-7.1, 49.8)
  line L18 (-7.1, 49.8) -> (-0.9, 49.8)
  line L19 (-0.9, 49.8) -> (-0.9, 56.1)
  circle A5 centre (-53, 53) radius 3.1
  line L20 (-53, 53) -> (-56.1, 53)
  line L21 (-56.1, 53) -> (-56.1, 56.1)
  line L22 (-56.1, 56.1) -> (-53, 56.1)
  line L23 (-53, 56.1) -> (-53, 53)
  line L24 (-56.1, 56.1) -> (-49.9, 56.1)
  line L25 (-49.9, 56.1) -> (-49.9, 49.8)
  line L26 (-49.9, 49.8) -> (-56.1, 49.8)
  line L27 (-56.1, 49.8) -> (-56.1, 56.1)
  dimension "d244" = 6.2
  dimension "d245" = 3.1
  dimension "d246" = 3.1
  dimension "d247" = 6.2
  dimension "d248" = 6.2
  dimension "d249" = 3.1
  dimension "d250" = 3.1
  dimension "d251" = 6.2
  constraint concentric A0 A4
  constraint horizontal L12
  constraint vertical L13
  constraint horizontal L14
  constraint vertical L15
  constraint coincident A0.centre A2.centre
  constraint horizontal L16
  constraint vertical L17
  constraint horizontal L18
  constraint vertical L19
  constraint concentric A1 A5
  constraint horizontal L20
  constraint vertical L21
  constraint horizontal L22
  constraint vertical L23
  constraint coincident A1.centre A3.centre
  constraint horizontal L24
  constraint vertical L25
  constraint horizontal L26
  constraint vertical L27
  measures "d244" diameter of A4
  measures "d245" distance of A0.centre L12.end
  measures "d246" distance of A0.centre L14.end
  measures "d247" distance of L13.end L16.end
  measures "d248" diameter of A5
  measures "d249" distance of A1.centre L20.end
  measures "d250" distance of A1.centre L22.end
  measures "d251" distance of L21.end L24.end
extrude "Extrude58" cut sketch "Sketch34" against normal blind 17 contours A0 A4 L12 L15 | A0 A4 L12 L15 | L10 A4 L17 L18 L19 | A4 L13 L14 L16 L19 | A4 L16 L17 | L6 A5 L25 L26 L27 | A1 A5 L20 L23 | A5 L24 L25 | A5 L21 L22 L24 L27 | A1 A5 L20 L23 | A1 L20 L23 | A1 L20 L23 bodies 3
sketch "Sketch35" plane through (-3.3, 0, 0) normal (-1, 0, 0) x (0, -1, 0)
  line L0 (0, 4) -> (0, 53)
  line L1 (0, 53) -> (-12.5, 53)
  line L2 (-12.5, 53) -> (-12.5, 4)
  line L3 (-12.5, 4) -> (0, 4)